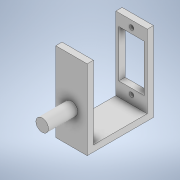
# Autodesk Inventor part: head_p2
Saved by Autodesk Inventor 2020.3 (Build 243373000, 373)
## iProperties
Created: 2020-08-24
Part Number: head_p2
Material: Generic
Document SubType Name: Modeling
Designer: aditk
Density: 1 g/cm^3
Appearance: Default
Author: aditk
Autodesk Inventor part; units mm, degrees
ref_plane "YZ Plane" through (0, 0, 0) normal (1, 0, 0) x (0, 1, 0)
ref_plane "XZ Plane" through (0, 0, 0) normal (0, 1, 0) x (-1, 0, 0)
ref_plane "XY Plane" through (0, 0, 0) normal (0, 0, 1) x (1, 0, 0)
sketch "Sketch1" plane through (0, 0, 0) normal (0, 1, 0) x (-1, 0, 0)
  line L0 (0, 15.85) -> (15, 15.85)
  line L1 (15, 15.85) -> (15, -15.85)
  line L2 (15, -15.85) -> (0, -15.85)
  line L3 (0, -15.85) -> (0, 15.85)
  point P0 (0, 0)
  constraints: 8 end point, 2 parallel, 1 horizontal, 1 perpendicular
extrude "Extrusion1" add sketch "Sketch1" along normal blind 3
sketch "Sketch2" plane through (0, 3, 0) normal (0, 1, 0) x (1, 0, 0)
  line L0 (-15, 15.85) -> (-15, -15.85) projected
  line L1 (0, -15.85) -> (0, 15.85) projected
  line L2 (-15, -15.85) -> (0, -15.85)
  line L3 (0, -15.85) -> (0, -12.85)
  line L4 (0, -12.85) -> (-15, -12.85)
  line L5 (-15, -12.85) -> (-15, -15.85)
  line L6 (0, 15.85) -> (-15, 15.85) projected
  line L7 (0, 15.85) -> (-15, 15.85)
  line L8 (-15, 15.85) -> (-15, 12.85)
  line L9 (-15, 12.85) -> (0, 12.85)
  line L10 (0, 12.85) -> (0, 15.85)
  point P0 (0, 0)
  dimension "d5" = 3
  dimension "d6" = 3
  constraints: 16 end point, 4 parallel, 2 horizontal, 2 perpendicular, 2 point on line
  measures "d5" distance of L3.end L2.end
  measures "d6" distance of L8.end L7.end
extrude "Extrusion2" add sketch "Sketch2" along normal blind 35 contours L6 L1 L9 L0 | L4 L1 L2 L0
sketch "Sketch4" plane through (0, 0, -15.85) normal (0, 0, -1) x (-1, 0, 0)
  arc A0 (8.05, 6.1974) -> (6.95, 6.1974) centre (7.5, 7.15) ccw
  line L0 (8.05, 5) -> (12.75, 5)
  line L1 (2.25, 5) -> (6.95, 5)
  line L2 (1.4, 10.65) -> (1.4, 5.85)
  line L3 (6.95, 37.1) -> (2.25, 37.1)
  line L4 (12.75, 37.1) -> (8.05, 37.1)
  arc A1 (6.95, 35.9026) -> (8.05, 35.9026) centre (7.5, 34.95) ccw
  line L5 (6.95, 37.1) -> (6.95, 35.9026)
  line L6 (8.05, 35.9026) -> (8.05, 37.1)
  line L7 (13.6, 31.45) -> (13.6, 36.25)
  line L8 (13.6, 5.85) -> (13.6, 10.65)
  arc A2 (12.75, 5) -> (13.6, 5.85) centre (12.75, 5.85) ccw
  line L9 (8.05, 5) -> (8.05, 6.1974)
  line L10 (6.95, 6.1974) -> (6.95, 5)
  arc A3 (1.4, 5.85) -> (2.25, 5) centre (2.25, 5.85) ccw
  arc A4 (2.25, 37.1) -> (1.4, 36.25) centre (2.25, 36.25) ccw
  line L11 (1.4, 36.25) -> (1.4, 31.45)
  line L12 (1.4, 27.762) -> (1.4, 31.45)
  line L13 (1.4, 10.65) -> (1.4, 24.638)
  circle A5 centre (7.5, 26.2) radius 2.25
  line L14 (13.6, 31.45) -> (13.6, 27.762)
  line L15 (13.6, 24.638) -> (13.6, 10.65)
  line L16 (2.25, 9.8) -> (12.75, 9.8)
  line L17 (12.75, 32.3) -> (2.25, 32.3)
  arc A6 (2.25, 32.3) -> (1.4, 31.45) centre (2.25, 31.45) ccw
  arc A7 (13.6, 31.45) -> (12.75, 32.3) centre (12.75, 31.45) ccw
  arc A8 (13.6, 36.25) -> (12.75, 37.1) centre (12.75, 36.25) ccw
  arc A9 (1.4, 10.65) -> (2.25, 9.8) centre (2.25, 10.65) ccw
  arc A10 (12.75, 9.8) -> (13.6, 10.65) centre (12.75, 10.65) ccw
  line L18 (13.6, 24.638) -> (13.6, 27.762)
  line L19 (1.4, 27.762) -> (1.4, 24.638)
  line L20 (0, 3) -> (15, 3) projected
  line L21 (15, 3) -> (0, 3)
  line L22 (0, 3) -> (0, 5)
  line L23 (0, 0) -> (0, 38) projected
  line L24 (0, 5) -> (15, 5)
  line L25 (15, 5) -> (15, 3)
  line L26 (15, 0) -> (15, 38) projected
  line L27 (7.5, 5) -> (7.5, 3)
  line L28 (8.05, 5) -> (6.95, 5)
  line L29 (7.5, 5) -> (7.5, 4.3316)
  line L30 (12.75, 37.1) -> (13.6, 37.1)
  line L31 (13.6, 37.1) -> (13.6, 36.25)
  line L32 (13.6, 5.85) -> (13.6, 5)
  line L33 (1.4, 5.85) -> (1.4, 5)
  line L34 (1.4, 36.25) -> (1.4, 37.1)
  line L35 (1.4, 37.1) -> (2.25, 37.1)
  line L36 (2.25, 32.3) -> (1.4, 32.3)
  line L37 (12.75, 32.3) -> (13.6, 32.3)
  line L38 (13.6, 10.65) -> (13.6, 9.8)
  line L39 (13.6, 9.8) -> (12.75, 9.8)
  line L40 (1.4, 9.8) -> (2.25, 9.8)
  circle A11 centre (7.5, 34.95) radius 1.1
  circle A12 centre (7.5, 7.15) radius 1.1
  point P0 (6.95, 6.1974)
  point P1 (8.05, 6.1974)
  point P2 (8.05, 35.9026)
  point P3 (6.95, 35.9026)
  dimension "d9" = 2
  constraints: 76 end point, 22 point on circle, 13 centre point, 11 point on line, 5 collinear, 3 midpoint, 3 perpendicular, 3 tangent, 2 coincident, 2 concentric, 2 horizontal, 1 vertical
  measures "d9" distance of L20.start L22.end
extrude "Extrusion3" cut sketch "Sketch4" against normal up to surface (3 mm away) contours A12 A0 | L39 A10 L8 | A10 L16 A9 L13 L19 L12 A6 L17 A7 L14 L18 L15 | L2 A9 L40 | A7 L37 L7 | L11 L36 A6 | A1 A11 | A5
sketch "Sketch6" plane through (-15, 0, 15.85) normal (0, 0, 1) x (1, 0, 0)
  circle A0 centre (7.5, 15.9) radius 3
  line L0 (0, 0) -> (0, 38)
  line L1 (0, 0) -> (15, 0)
  line L2 (15, 0) -> (15, 38)
  constraints: 6 end point, 1 centre point
extrude "Extrusion5" add sketch "Sketch6" along normal blind 14
body "Solid1"
